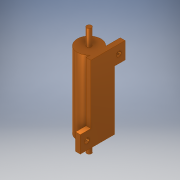
# Autodesk Inventor part: Power Resistor - HSA50
Saved by Autodesk Inventor 2017 (Build 210142000, 142)
## iProperties
Created: 2022-12-04
Part Number: Power Resistor - HSA50
Material: Gold
Document SubType Name: Modeling
Designer: Win240
Mass: 273.3 g
Surface Area: 53.5113 cm^2
Volume: 14.1606 cm^3
Density: 19.3 g/cm^3
Appearance: Metal 1600F Hot
Author: Win240
Autodesk Inventor part; units mm, degrees
ref_plane "YZ Plane" through (0, 0, 0) normal (1, 0, 0) x (0, 1, 0)
ref_plane "XZ Plane" through (0, 0, 0) normal (0, 1, 0) x (-1, 0, 0)
ref_plane "XY Plane" through (0, 0, 0) normal (0, 0, 1) x (1, 0, 0)
sketch "Sketch1" plane through (0, 0, 0) normal (0, 1, 0) x (-1, 0, 0)
  arc A0 (3.2, -5.2536) -> (17, 0) centre (9.1, 0) ccw
  line L0 (3.2, -5.2536) -> (3.2, -15)
  line L1 (3.2, -15) -> (0, -15)
  line L2 (0, -15) -> (0, 15)
  line L3 (0, 15) -> (3.2, 15)
  line L4 (3.2, 15) -> (3.2, 5.2536)
  arc A1 (17, 0) -> (3.2, 5.2536) centre (9.1, 0) ccw
  line L5 (9.1, 7.9) -> (9.1, -7.9) construction
  line L6 (3.2, 5.2536) -> (17, 0) construction
  line L7 (3.2, -5.2536) -> (17, 0) construction
  point P0 (0, 0)
  point P1 (0, 0)
  dimension "d0" = 3.2
  dimension "d1" = 30
  dimension "d5" = 15.8
  dimension "d6" = 17
  constraints: 16 end point, 6 point on circle, 4 vertical, 3 equal length, 2 centre point, 2 concentric, 2 horizontal, 2 line through centre, 1 coincident, 1 midpoint
  measures "d0" distance of L0.end L1.end
  measures "d1" distance of L1.end L2.end
  measures "d5" distance of L5.start L5.end
  measures "d6" distance from line of L6.end L2
extrude "Extrusion1" add sketch "Sketch1" along normal blind 51
sketch "Sketch2" plane through (0, 0, 15) normal (1, 0, 0) x (0, 0, -1)
  circle A0 centre (25.7, 45.35) radius 1.65
  circle A1 centre (4.3, 5.65) radius 1.65
  line L0 (25.7, 45.35) -> (25.7, 5.65) construction
  line L1 (25.7, 5.65) -> (4.3, 5.65) construction
  line L2 (30, 0) -> (30, 51) projected
  line L3 (0, 0) -> (0, 51) projected
  line L4 (25.7, 45.35) -> (30, 45.35) construction
  line L5 (25.7, 45.35) -> (30, 51) construction
  line L6 (0, 0) -> (4.3, 5.65) construction
  line L7 (4.3, 5.65) -> (0, 5.65) construction
  line L8 (30, 39.7) -> (22.9, 39.7)
  line L9 (22.9, 39.7) -> (22.9, 0)
  line L10 (22.9, 0) -> (30, 0)
  line L11 (0, 11.3) -> (7.1, 11.3)
  line L12 (7.1, 11.3) -> (7.1, 51)
  line L13 (7.1, 51) -> (0, 51)
  line L14 (25.7, 45.35) -> (30, 39.7) construction
  point P0 (15, 0)
  dimension "d9" = 21.4
  dimension "d10" = 39.7
  dimension "d11" = 3.3
  dimension "d12" = 2.8
  constraints: 26 end point, 7 horizontal, 5 equal length, 4 point on line, 3 vertical, 2 centre point, 1 equal radius
  measures "d9" distance of L0.end L1.end
  measures "d10" distance of L0.start L0.end
  measures "d11" diameter of A0
  measures "d12" distance from line of L0.start L9
extrude "Extrusion2" cut sketch "Sketch2" against normal up to surface (3.2 mm away)
sketch "Sketch3" plane through (0, 0, 0) normal (0, -1, 0) x (1, 0, 0)
  arc A0 (-3.2, 5.2536) -> (-3.2, -5.2536) centre (-9.1, 0) ccw projected
  circle A1 centre (-9.1, 0) radius 1.5875
  point P0 (0, 0)
  dimension "d15" = 3.175
  constraints: 1 centre point, 1 coincident
  measures "d15" diameter of A1
extrude "Extrusion3" add sketch "Sketch3" along normal blind 11
sketch "Sketch4" plane through (0, 51, 0) normal (0, 1, 0) x (1, 0, 0)
  arc A0 (-3.2, 5.2536) -> (-3.2, -5.2536) centre (-9.1, 0) ccw construction
  circle A1 centre (-9.1, 0) radius 1.5875
  point P0 (0, 0)
  dimension "d18" = 3.175
  constraints: 1 centre point, 1 coincident
  measures "d18" diameter of A1
extrude "Extrusion4" add sketch "Sketch4" along normal blind 11
body "Solid1"
